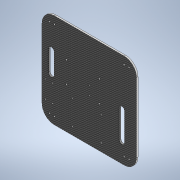
# Autodesk Inventor part: payload_bay_square_drill_holes
Saved by Autodesk Inventor 2020.2 (Build 242310000, 310)
## iProperties
Created: 2020-02-19
Part Number: payload_bay_square_drill_holes
Material: Generic
Document SubType Name: Modeling
Designer: Krishna Makhija
Density: 1 g/cm^3
Appearance: Default
Author: Krishna Makhija
Autodesk Inventor part; units mm, degrees
ref_plane "YZ Plane" through (0, 0, 0) normal (1, 0, 0) x (0, 1, 0)
ref_plane "XZ Plane" through (0, 0, 0) normal (0, 1, 0) x (-1, 0, 0)
ref_plane "XY Plane" through (0, 0, 0) normal (0, 0, 1) x (1, 0, 0)
sketch "Sketch1" plane through (0, 0, 0) normal (0, 0, 1) x (1, 0, 0)
  point P0 (0, 0)
sketch "Sketch2" plane through (0, 0, 0) normal (0, 0, 1) x (1, 0, 0)
  line L0 (94.9998, -95.0001) -> (-94.9998, -95.0001)
  line L1 (-94.9998, -95.0001) -> (-94.9998, 95.0001)
  line L2 (-94.9998, 95.0001) -> (94.9998, 95.0001)
  line L3 (94.9998, 95.0001) -> (94.9998, -95.0001)
  line L4 (94.9998, -95.0001) -> (-94.9998, 95.0001) construction
  line L5 (-94.9998, -95.0001) -> (94.9998, 95.0001) construction
  point P0 (0, 0)
  constraints: 12 end point, 2 midpoint, 2 parallel, 1 horizontal, 1 perpendicular
extrude "Extrusion1" add sketch "Sketch2" along normal blind 3
sketch "Sketch3" plane through (0, 0, 3) normal (0, 0, 1) x (1, 0, 0)
  circle A0 centre (70, 80) radius 1.5001
  circle A1 centre (70, -80) radius 1.5001
  circle A2 centre (-70, 80) radius 1.5001
  circle A3 centre (-70, -80) radius 1.5001
  constraints: 4 centre point
extrude "Extrusion2" cut sketch "Sketch3" against normal blind 3
fillet "Fillet1" radius 25 1 edges at (94.9998, 95.0001, 1.5)
fillet "Fillet2" radius 25 1 edges at (94.9998, -95.0001, 1.5)
fillet "Fillet3" radius 25 1 edges at (-94.9998, -95.0001, 1.5)
fillet "Fillet4" radius 25 1 edges at (-94.9998, 95.0001, 1.5)
sketch "Pi mount holes" plane through (0, 0, 3) normal (0, 0, 1) x (1, 0, 0)
  circle A0 centre (24, -30.5) radius 1.2502
  circle A1 centre (-34, -30.5) radius 1.2502
  circle A2 centre (-34, -79.5) radius 1.2502
  circle A3 centre (24, -79.5) radius 1.2502
  constraints: 4 centre point
sketch "B205 mount holes" plane through (0, 0, 3) normal (0, 0, 1) x (1, 0, 0)
  circle A0 centre (20.32, 30.48) radius 1.5002
  circle A1 centre (-45.72, 30.48) radius 1.5002
  circle A2 centre (-45.72, -12.7) radius 1.5002
  circle A3 centre (20.32, -12.7) radius 1.5002
  constraints: 4 centre point
sketch "RM3100 mount holes" plane through (0, 0, 3) normal (0, 0, 1) x (1, 0, 0)
  circle A0 centre (0, 9) radius 0.9999
  circle A1 centre (0, -9) radius 0.9999
  constraints: 2 centre point
sketch "Pololu mount holes" plane through (0, 0, 3) normal (0, 0, 1) x (1, 0, 0)
  circle A0 centre (-73.2965, -23.9932) radius 1.1973
  circle A1 centre (-88.2965, -23.9932) radius 1.1973
  circle A2 centre (-73.2965, -59.4932) radius 1.1973
  circle A3 centre (-88.2965, -59.4932) radius 1.1973
  constraints: 4 centre point
sketch "B205 cable cutout" plane through (0, 0, 3) normal (0, 0, 1) x (1, 0, 0)
  line L0 (-76.0426, -14.5593) -> (-76.0426, 37.4411) construction
  line L1 (-81.5424, -9.0595) -> (-81.5424, 31.9413)
  line L2 (-70.5428, 31.9413) -> (-70.5428, -9.0595)
  arc A0 (-81.5424, -9.0595) -> (-70.5428, -9.0595) centre (-76.0426, -9.0595) ccw
  arc A1 (-70.5428, 31.9413) -> (-81.5424, 31.9413) centre (-76.0426, 31.9413) ccw
  point P0 (0, 0)
  point P1 (-76.0426, 11.4409)
  constraints: 8 end point, 6 point on circle, 4 tangent, 2 centre point, 2 point on line, 1 midpoint, 1 parallel, 1 vertical
sketch "Pi cable cutout" plane through (0, 0, 3) normal (0, 0, 1) x (1, 0, 0)
  line L0 (65.7382, -60.7056) -> (65.7382, 5.2939) construction
  line L1 (60.7378, -55.7052) -> (60.7378, 0.2935)
  line L2 (70.7387, 0.2935) -> (70.7387, -55.7052)
  arc A0 (60.7378, -55.7052) -> (70.7387, -55.7052) centre (65.7382, -55.7052) ccw
  arc A1 (70.7387, 0.2935) -> (60.7378, 0.2935) centre (65.7382, 0.2935) ccw
  point P0 (0, 0)
  point P1 (65.7382, -27.7058)
  constraints: 8 end point, 6 point on circle, 4 tangent, 2 centre point, 2 point on line, 1 midpoint, 1 parallel, 1 vertical
sketch "Imperial standoffs" plane through (0, 0, 3) normal (0, 0, 1) x (1, 0, 0)
  circle A0 centre (80, 80) radius 1.4302
  circle A1 centre (-80, -80) radius 1.4302
  circle A2 centre (80, -80) radius 1.4302
  circle A3 centre (-80, 80) radius 1.4302
  constraints: 4 centre point
extrude "Extrusion3" cut sketch "B205 cable cutout" against normal blind 10
extrude "Extrusion4" cut sketch "Pi cable cutout" against normal blind 10
extrude "Extrusion5" cut sketch "Imperial standoffs" against normal blind 10
extrude "Extrusion6" cut sketch "Pololu mount holes" against normal blind 10
extrude "Extrusion7" cut sketch "B205 mount holes" against normal blind 10
extrude "Extrusion8" cut sketch "RM3100 mount holes" against normal blind 10
extrude "Extrusion9" cut sketch "Pi mount holes" against normal blind 10
body "Solid1"
